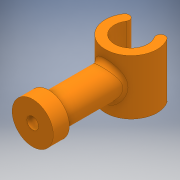
# Autodesk Inventor part: Laser Mount
Saved by Autodesk Inventor 2018 (Build 220112000, 112)
## iProperties
Created: 2018-01-13
Part Number: Laser Mount
Material: Generic
Document SubType Name: Modeling
Designer: Moochster
Density: 1 g/cm^3
Appearance: Orange
Mass: 1.0836 g
Surface Area: 11.8394 cm^2
Volume: 1.0836 cm^3
Author: Moochster
Autodesk Inventor part; units mm, degrees
ref_plane "YZ Plane" through (0, 0, 0) normal (1, 0, 0) x (0, 1, 0)
ref_plane "XZ Plane" through (0, 0, 0) normal (0, 1, 0) x (-1, 0, 0)
ref_plane "XY Plane" through (0, 0, 0) normal (0, 0, 1) x (1, 0, 0)
sketch "Sketch1" plane through (0, 0, 0) normal (0, 1, 0) x (-1, 0, 0)
  circle A0 centre (0, 0) radius 1.125 construction
  circle A1 centre (0, 0) radius 1.275
  circle A2 centre (0, 0) radius 4.5
  dimension "d1" = 2.25
  dimension "d2" = 0.15
  dimension "d3" = 9
  constraints: 3 centre point, 3 coincident
  measures "d1" diameter of A0
  measures "d2" radial gap between concentric circles of A0 A1
  measures "d3" diameter of A2
extrude "Extrusion1" add sketch "Sketch1" along normal blind 3.5
sketch "Sketch2" plane through (0, 3.5, 0) normal (0, 1, 0) x (1, 0, 0)
  circle A0 centre (0, 0) radius 1.275 projected
  circle A1 centre (0, 0) radius 3.275
  dimension "d6" = 2
  constraints: 1 centre point
  measures "d6" radial gap between concentric circles of A0 A1
extrude "Extrusion2" add sketch "Sketch2" along normal blind 18
sketch "Sketch3" plane through (0, 0, 0) normal (0, 0, 1) x (1, 0, 0)
  line L0 (3.275, 21.5) -> (-3.275, 21.5) projected
  line L1 (-1.275, 21.5) -> (1.275, 21.5) projected
  circle A0 centre (0, 21.5) radius 3.65
  circle A1 centre (0, 21.5) radius 5.65
  line L2 (3.9952, 25.4952) -> (2.5809, 24.0809)
  line L3 (-2.5809, 24.0809) -> (-3.9952, 25.4952)
  line L4 (2.5809, 24.0809) -> (-2.5809, 24.0809) construction
  point P0 (0, 0)
  point P1 (0, 24.0809)
  dimension "d9" = 7.3
  dimension "d10" = 2
  constraints: 6 end point, 4 point on circle, 3 midpoint, 2 centre point, 2 line through centre, 1 coincident, 1 horizontal, 1 perpendicular, 1 vertical alignment
  measures "d9" diameter of A0
  measures "d10" radial gap between concentric circles of A0 A1
extrude "Extrusion3" cut sketch "Sketch3" along normal through all both and the other way through all contours A0 | A0 L2 A1 L3 picked at (-3.9907, 24.4254)
extrude "Extrusion4" add sketch "Sketch3" along normal mid plane 12 contours A0 L2 A1 L3 picked at (-3.9907, 24.4254)
fillet "Fillet1" radius 1 4 edges at (-2.5809, 24.0809, 0) (2.5809, 24.0809, 0) (-3.9952, 25.4952, 0) (3.9952, 25.4952, 0)
fillet "Fillet2" radius 1 1 edges at (-3.275, 16.896, -0.0035)
body "Solid1"
